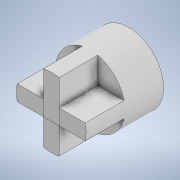
# Autodesk Inventor part: 3xxx_Tx_Coil_Winding_MPSv2_v1.form
Saved by Autodesk Inventor 2021 (Build 250183000, 183)
## iProperties
Created: 2020-09-17
Part Number: 3xxx_Tx_Coil_Winding_MPSv2_v1.form
Material: Generic
Document SubType Name: Modeling
Designer: Admin
Density: 1 g/cm^3
Appearance: Default
Author: Admin
Autodesk Inventor part; units mm, degrees
ref_plane "YZ Plane" through (0, 0, 0) normal (1, 0, 0) x (0, 1, 0)
ref_plane "XZ Plane" through (0, 0, 0) normal (0, 1, 0) x (-1, 0, 0)
ref_plane "XY Plane" through (0, 0, 0) normal (0, 0, 1) x (1, 0, 0)
sketch "Sketch1" plane through (0, 0, 0) normal (0, 0, 1) x (1, 0, 0)
  circle A0 centre (0, 0) radius 22.5
  arc A1 (7.2901, 17.5999) -> (-7.2901, 17.5999) centre (0, 0) ccw
  line L0 (-7.2901, 17.5999) -> (-7.5205, 17.5027)
  line L1 (-4.7835, 11.5485) -> (-4.8792, 11.7795)
  line L2 (-7.5205, 17.5027) -> (-4.7835, 11.0159)
  line L3 (-11.5485, 4.7835) -> (-11.7795, 4.8792)
  line L4 (-11.7795, 4.8792) -> (-4.8792, 11.7795)
  line L5 (0, 0) -> (-3.3576, 3.3576)
  line L6 (0, 0) -> (0, 3.3576)
  line L7 (0, 0) -> (-2.7445, 0)
  line L8 (-17.5027, 7.5205) -> (-11.0159, 4.7835)
  line L9 (0, 0) -> (2.6435, 2.6435)
  line L10 (7.5205, -17.5027) -> (4.7835, -11.0159)
  line L11 (4.8792, -11.7795) -> (11.7795, -4.8792)
  line L12 (17.5027, -7.5205) -> (11.0159, -4.7835)
  line L13 (17.5027, 7.5205) -> (11.0159, 4.7835)
  line L14 (11.7795, 4.8792) -> (4.8792, 11.7795)
  line L15 (7.5205, 17.5027) -> (4.7835, 11.0159)
  line L16 (-17.5027, -7.5205) -> (-11.0159, -4.7835)
  line L17 (-11.7795, -4.8792) -> (-4.8792, -11.7795)
  line L18 (-7.5205, -17.5027) -> (-4.7835, -11.0159)
  arc A2 (-17.5027, 7.5205) -> (-17.5027, -7.5205) centre (0, 0) ccw
  arc A3 (-7.5205, -17.5027) -> (7.5205, -17.5027) centre (0, 0) ccw
  arc A4 (17.5027, -7.5205) -> (17.5027, 7.5205) centre (0, 0) ccw
  arc A5 (7.5205, 17.5027) -> (-7.5205, 17.5027) centre (0, 0) ccw
  line L19 (17.5027, 7.5205) -> (18.4489, 7.9197)
  line L20 (7.5205, 17.5027) -> (7.9197, 18.4489)
  line L21 (-17.5027, 7.5205) -> (-18.4489, 7.9197)
  line L22 (-7.5205, 17.5027) -> (-7.9197, 18.4489)
  line L23 (17.5027, -7.5205) -> (18.4489, -7.9197)
  line L24 (7.5205, -17.5027) -> (7.9197, -18.4489)
  line L25 (-7.5205, -17.5027) -> (-7.9197, -18.4489)
  line L26 (-17.5027, -7.5205) -> (-18.4489, -7.9197)
  arc A6 (7.5496, 17.5718) -> (-7.5496, 17.5718) centre (0, 0) ccw
  arc A7 (17.5718, -7.5496) -> (17.5718, 7.5496) centre (0, 0) ccw
  arc A8 (-17.5718, 7.5496) -> (-17.5718, -7.5496) centre (0, 0) ccw
  arc A9 (-7.5496, -17.5718) -> (7.5496, -17.5718) centre (0, 0) ccw
  point P0 (-5.0385, -11.6202)
  point P1 (-11.6202, -5.0385)
  point P2 (-11.6202, 5.0385)
  point P3 (-5.0385, 11.6202)
  point P4 (5.0385, 11.6202)
  point P5 (11.6202, 5.0385)
  point P6 (11.6202, -5.0385)
  point P7 (5.0385, -11.6202)
  dimension "d0" = 45
  dimension "d1" = 0.25
  dimension "d2" = 0.25
  dimension "d3" = 0.25
  constraints: 54 end point, 27 symmetric about line, 18 point on circle, 10 centre point, 8 point on line, 3 coincident, 1 horizontal, 1 vertical
  measures "d0" diameter of A0
  measures "d1" distance of L0.start L0.end
  measures "d2" distance of L1.start L1.end
  measures "d3" distance of L3.start L3.end
extrude "Extrusion1" add sketch "Sketch1" along normal blind 20
sketch "Sketch2" plane through (0, 0, 20) normal (0, 0, 1) x (1, 0, 0)
  circle A0 centre (13.946, 0) radius 2.875
  circle A1 centre (0, -13.946) radius 2.875
  circle A2 centre (-13.946, 0) radius 2.875
  circle A3 centre (0, 13.946) radius 2.875
  point P0 (0, 0)
  point P1 (0, 0)
  dimension "d7" = 5.75
  dimension "d8" = 5.75
  dimension "d9" = 5.75
  dimension "d10" = 5.75
  constraints: 4 centre point
  measures "d7" diameter of A0
  measures "d8" diameter of A1
  measures "d9" diameter of A2
  measures "d10" diameter of A3
extrude "Extrusion2" add sketch "Sketch2" against normal blind 5
sketch "Sketch3" plane through (0, 0, 20) normal (0, 0, 1) x (1, 0, 0)
  circle A0 centre (0, 0) radius 22.5
  constraints: 1 centre point, 1 coincident
extrude "Extrusion3" add sketch "Sketch3" along normal blind 5
sketch "Sketch4" plane through (0, 0, 25) normal (0, 0, 1) x (1, 0, 0)
  line L0 (-5, -5) -> (5, -5)
  line L1 (5, -5) -> (5, 5)
  line L2 (5, 5) -> (-5, 5)
  line L3 (-5, 5) -> (-5, -5)
  line L4 (-5, -5) -> (5, 5) construction
  line L5 (5, -5) -> (-5, 5) construction
  circle A0 centre (0, 0) radius 22.5 projected
  line L6 (5, 5) -> (-3.5794, 5)
  line L7 (5, 5) -> (-5, 5)
  line L8 (-5, 5) -> (-5, 25)
  line L9 (-5, 25) -> (5, 25)
  line L10 (5, 25) -> (5, 5)
  line L11 (-4.9693, -4.9693) -> (-24.9693, -4.9693)
  line L12 (-24.9693, -4.9693) -> (-24.9693, 5.0307)
  line L13 (-24.9693, 5.0307) -> (-4.9693, 5.0307)
  line L14 (-4.9693, 5.0307) -> (-4.9693, -4.9693)
  line L15 (-4.9693, -4.9693) -> (5.0307, -4.9693)
  line L16 (5.0307, -4.9693) -> (5.0307, -24.9693)
  line L17 (5.0307, -24.9693) -> (-4.9693, -24.9693)
  line L18 (-4.9693, -24.9693) -> (-4.9693, -4.9693)
  line L19 (5.0307, -4.9693) -> (25.0307, -4.9693)
  line L20 (25.0307, -4.9693) -> (25.0307, 5.0307)
  line L21 (25.0307, 5.0307) -> (5.0307, 5.0307)
  line L22 (5.0307, 5.0307) -> (5.0307, -4.9693)
  circle A1 centre (0, 0) radius 22.5
  point P0 (-4.9693, -5)
  point P1 (-4.9693, -21.9444)
  point P2 (5.0307, -21.9304)
  point P3 (5, -4.9693)
  point P4 (-5, 5.0307)
  point P5 (-21.9304, 5.0307)
  point P6 (-21.9444, -4.9693)
  point P7 (-5, -4.9693)
  point P8 (5, 21.9374)
  point P9 (-5, 21.9374)
  point P10 (21.9444, -4.9693)
  point P11 (21.9304, 5.0307)
  dimension "d15" = 10
  dimension "d16" = 10
  dimension "d17" = 10
  dimension "d18" = 20
  dimension "d19" = 20
  dimension "d20" = 10
  dimension "d21" = 10
  dimension "d22" = 20
  dimension "d23" = 20
  dimension "d24" = 10
  constraints: 46 end point, 10 parallel, 6 horizontal, 5 perpendicular, 2 midpoint, 1 centre point, 1 coincident, 1 concentric
  measures "d15" distance of L2.end L1.end
  measures "d16" distance of L1.end L0.end
  measures "d17" distance of L8.end L9.end
  measures "d18" distance of L7.end L8.end
  measures "d19" distance of L12.end L13.end
  measures "d20" distance of L11.end L12.end
  measures "d21" distance of L16.end L17.end
  measures "d22" distance of L15.end L16.end
  measures "d23" distance of L21.end L20.end
  measures "d24" distance of L20.end L19.end
extrude "Extrusion4" add sketch "Sketch4" along normal blind 25 contours L0 L1 L15 L16 A0 L18 | L11 A0 L13 L8 L3 | L14 L2 L1 L15 | L14 L13 L8 A0 L10 L2 | L22 L21 A0 L19
body "Solid1"
